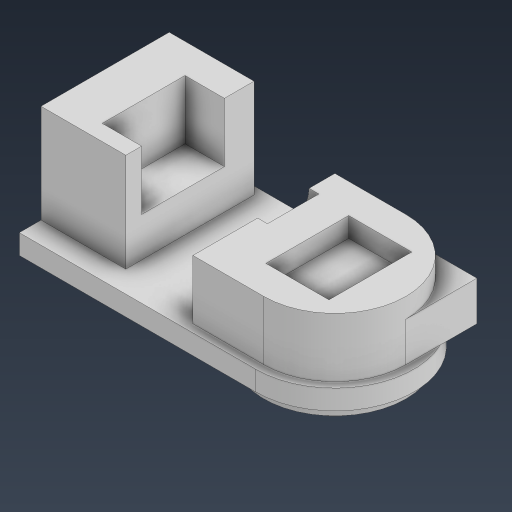
# Autodesk Inventor part: Axis1
Saved by Autodesk Inventor 2024 (Build 280153000, 153)
## iProperties
Created: 2025-08-29
Part Number: Axis1
Material: Generic
Document SubType Name: Modeling
Designer: Piter
Density: 1 g/cm^3
Appearance: Default
Author: Piter
Autodesk Inventor part; units mm, degrees
ref_plane "YZ Plane" through (0, 0, 0) normal (1, 0, 0) x (0, 1, 0)
ref_plane "XZ Plane" through (0, 0, 0) normal (0, 1, 0) x (-1, 0, 0)
sketch "Sketch1" plane through (0, 0, 0) normal (0, 1, 0) x (-1, 0, 0)
  circle A0 centre (0, 0) radius 19.95
  dimension "d0" = 39.9
  constraints: 1 centre point, 1 coincident
  measures "d0" diameter of A0
extrude "Extrusion1" add sketch "Sketch1" along normal blind 11.5
sketch "Sketch3" plane through (0, 11.5, 0) normal (0, 1, 0) x (1, 0, 0)
  circle A0 centre (0, 0) radius 36
  dimension "d4" = 72
  constraints: 1 centre point, 1 coincident
  measures "d4" diameter of A0
extrude "Extrusion2" add sketch "Sketch3" along normal blind 5
sketch "Sketch5" plane through (0, 0, 0) normal (0, -1, 0) x (1, 0, 0)
  circle A0 centre (0, 0) radius 12
  dimension "d10" = 24
  constraints: 1 centre point, 1 coincident
  measures "d10" diameter of A0
extrude "Extrusion4" add sketch "Sketch5" along normal blind 4
sketch "Sketch6" plane through (0, -4, 0) normal (0, -1, 0) x (1, 0, 0)
  circle A0 centre (0, 0) radius 8
  dimension "d13" = 16
  constraints: 1 centre point, 1 coincident
  measures "d13" diameter of A0
extrude "Extrusion5" cut sketch "Sketch6" against normal blind 7
sketch "Sketch7" plane through (0, 0, 0) normal (0, 0, 1) x (1, 0, 0)
  line L0 (-12, -4) -> (12, -4) projected
  line L1 (0, -4) -> (0, 16.5) construction
  line L2 (36, 16.5) -> (-36, 16.5) projected
  circle A0 centre (0, -0.5) radius 2.05
  point P0 (0, 0)
  dimension "d16" = 4.1
  dimension "d17" = 3.5
  constraints: 2 end point, 2 midpoint, 1 centre point, 1 point on line
  measures "d16" diameter of A0
  measures "d17" distance from line of L0 A0.centre
extrude "Extrusion6" cut sketch "Sketch7" against normal through all
ref_plane "Work Plane1" through (0, 0, -9) normal (0, 0, 1) x (1, 0, 0)
sketch "Sketch8" plane through (0, 0, -9) normal (0, 0, 1) x (1, 0, 0)
  spline S0 degree 8 poles (2.05, -0.5) (2.05, -0.2848) (2.0242, -0.07) (1.9727, 0.1426) (1.8952, 0.3508) (1.7908, 0.5524) (1.6587, 0.744) (1.4975, 0.9217) (1.1428, 1.2152) (0.9502, 1.3418) (0.7319, 1.4481) (0.4932, 1.5258) (0.2416, 1.5696) (-0.015, 1.5768) (-0.268, 1.5477) (-0.7585, 1.4217) (-0.9865, 1.3253) (-1.1913, 1.203) (-1.372, 1.0604) (-1.5283, 0.9024) (-1.6604, 0.7329) (-1.769, 0.5554) (-1.9523, 0.1659) (-2.022, -0.0509) (-2.064, -0.2739) (-2.0779, -0.5) (-2.064, -0.7261) (-2.022, -0.9491) (-1.9523, -1.1659) (-1.7743, -1.544) (-1.674, -1.7105) (-1.5532, -1.8699) (-1.4114, -2.0197) (-1.2482, -2.1567) (-1.0637, -2.2771) (-0.8583, -2.3766) (-0.4199, -2.5191) (-0.1917, -2.5636) (0.0445, -2.5784) (0.2816, -2.5615) (0.512, -2.5135) (0.7285, -2.4379) (0.9254, -2.3407) (1.3434, -2.0754) (1.5505, -1.8884) (1.7199, -1.6798) (1.8532, -1.4566) (1.9518, -1.2237) (2.0171, -0.9848) (2.05, -0.7427) (2.05, -0.5) knots 0 0 0 0 0 0 0 0 0 0.154447 0.154447 0.154447 0.154447 0.154447 0.154447 0.154447 0.287129 0.287129 0.287129 0.287129 0.287129 0.287129 0.287129 0.423569 0.423569 0.423569 0.423569 0.423569 0.423569 0.423569 0.578272 0.578272 0.578272 0.578272 0.578272 0.578272 0.578272 0.706239 0.706239 0.706239 0.706239 0.706239 0.706239 0.706239 0.827838 0.827838 0.827838 0.827838 0.827838 0.827838 0.827838 1 1 1 1 1 1 1 1 1 projected
  line L0 (8, 3) -> (-8, 3) projected
  line L1 (8, -4) -> (-8, -4) projected
  circle A0 centre (0, -0.5) radius 3
  point P0 (0, 0)
  dimension "d21" = 6
  constraints: 1 centre point, 1 other
  measures "d21" diameter of A0
extrude "Extrusion7" cut sketch "Sketch8" against normal through all
pattern_circular "Circular Pattern1" count 2 over 90 about axis through (0, -10, 0) along (0, 1, 0) of "Extrusion7", "Extrusion6"
sketch "Sketch10" plane through (0, 16.5, 0) normal (0, 1, 0) x (1, 0, 0)
  circle A0 centre (0, 0) radius 36 projected
  circle A1 centre (0, 0) radius 40
  line L0 (0, 40) -> (0, -40)
  line L1 (0, -40) -> (-70, -40)
  line L2 (-70, -40) -> (-70, 40)
  line L3 (-70, 40) -> (0, 40)
  dimension "d51" = 80
  dimension "d67" = 70
  constraints: 8 end point, 2 parallel, 2 point on circle, 1 centre point, 1 coincident, 1 perpendicular
  measures "d51" diameter of A1
  measures "d67" distance of L0.end L1.end
extrude "Extrusion8" add sketch "Sketch10" along normal blind 10 contours A0 L0 | A0 L0 A1 | L0 A0 | A0 L0 A1
sketch "Sketch11" plane through (0, 26.5, 0) normal (0, 1, 0) x (1, 0, 0)
  line L0 (-36, -36) -> (36, -36)
  line L1 (36, -36) -> (36, 36)
  line L2 (36, 36) -> (-36, 36)
  line L3 (-36, 36) -> (-36, -36)
  circle A0 centre (0, 0) radius 8 projected
  line L4 (-36, -36) -> (36, 36) construction
  line L5 (36, -36) -> (-36, 36) construction
  line L6 (0, 36) -> (0, -36) construction
  line L7 (-36, 0) -> (36, 0) construction
  circle A1 centre (0, 0) radius 36 projected
  line L8 (-14, -21) -> (18, -21)
  line L9 (18, -21) -> (18, 21)
  line L10 (18, 21) -> (-14, 21)
  line L11 (-14, 21) -> (-14, -21)
  line L12 (-14, -21) -> (18, 21) construction
  line L13 (18, -21) -> (-14, 21) construction
  circle A2 centre (0, 0) radius 40 projected
  line L14 (18, 21) -> (18, 35.7211)
  line L15 (18, -21) -> (18, -35.7211)
  line L16 (18, 35.7211) -> (18, -35.7211)
  line L17 (18, -35.7211) -> (-34, -35.7211)
  line L18 (-34, -35.7211) -> (-34, 35.7211)
  line L19 (-34, 35.7211) -> (18, 35.7211)
  line L20 (-14, 0) -> (-36, 0)
  line L21 (18, -29) -> (-21.3307, -29)
  point P0 (2, 0)
  point P1 (-18, 35.7211)
  point P2 (-36, 29.3939)
  point P3 (-36, -29.3939)
  point P4 (-18, -35.7211)
  point P5 (6, -5.2915)
  point P6 (6, 5.2915)
  point P7 (6, 36)
  point P8 (6, -36)
  point P9 (18, -29)
  point P10 (18, 31.1769)
  point P11 (18, -31.1769)
  dimension "d35" = 72
  dimension "d36" = 72
  dimension "d37" = 32
  dimension "d38" = 42
  dimension "d39" = 18
  dimension "d40" = 52
  dimension "d53" = 7
  constraints: 44 end point, 9 midpoint, 6 parallel, 4 perpendicular, 4 point on circle, 3 point on line, 2 horizontal, 1 collinear, 1 vertical
  measures "d35" distance of L2.end L1.end
  measures "d36" distance of L1.end L0.end
  measures "d37" distance of L10.end L9.end
  measures "d38" distance of L9.end L8.end
  measures "d39" distance between parallel lines of L1 L9
  measures "d40" distance of L15.end L17.end
  measures "d53" distance between parallel lines of L0 L21
extrude "Extrusion9" add sketch "Sketch11" along normal blind 20 contours L3 A2 L18 L17 L0 | A2 L17 A1 L0 | L3 A1 L18 A2 | A1 L17 A2 L0 | A1 L17 | L17 L18 A2 | A2 L18 A1 L17 | A2 L1 L0 | L3 A2 L18 A1 | L20 L18 A1 | A1 L18 L20 | L3 L2 A2 L19 L18 | A1 L21 L15 L17 | A1 L15 L17 | L15 A1 L1 A2 | L18 A2 L19 A1 | A1 L19 L14 L10 L11 L20 L18 | L18 L20 L11 L8 L15 L21 A1 | L18 L19 A2 | L15 L9 L14 A1 | L19 A2 L2 A1 | A1 L19 | L11 L10 L9 L8 | A1 L14 A2 L1 | L2 A2 L19 A1 | L19 L14 A1 | L2 L1 A2 | A0
extrude "Extrusion10" add sketch "Sketch11" along normal blind 30 contours L3 A2 L18 L17 L0 | A2 L17 A1 L0 | L3 A1 L18 A2 | A1 L17 | L17 L18 A2 | A2 L18 A1 L17 | L3 A2 L18 A1 | L20 L18 A1 | A1 L18 L20 | L3 L2 A2 L19 L18 | A1 L21 L15 L17 | L18 A2 L19 A1 | A1 L19 L14 L10 L11 L20 L18 | L18 L20 L11 L8 L15 L21 A1 | L18 L19 A2 | L15 L9 L14 A1 | L19 A2 L2 A1 | A1 L19 picked at (-8.298, -35.8657) picked at (-8.298, 35.8657)
sketch "Sketch15" plane through (0, 46.5, 0) normal (0, 1, 0) x (1, 0, 0)
  arc A0 (0, -36) -> (36, 0) centre (0, 0) ccw projected
  line L0 (0, -36) -> (36, -36) projected
  line L1 (36, -36) -> (36, 0) projected
  arc A1 (36, 0) -> (0, 36) centre (0, 0) ccw projected
  line L2 (36, 0) -> (36, 36) projected
  line L3 (36, 36) -> (0, 36) projected
extrude "Extrusion12" cut sketch "Sketch15" against normal up to surface (20 mm away) contours A0 L1 L0
sketch "Sketch16" plane through (0, 56.5, 0) normal (0, 1, 0) x (1, 0, 0)
  line L0 (-14, -21) -> (-14, 21) projected
  line L1 (18, -21) -> (-14, -21) projected
  line L2 (-14, -21) -> (-14, 21) projected
  line L3 (-14, 21) -> (18, 21) projected
  line L4 (0, 36) -> (-36, 36) projected
  line L5 (-36, 36) -> (-36, -36) projected
  arc A0 (0, -36) -> (0, 36) centre (0, 0) ccw projected
  line L6 (-34.5832, -10) -> (-14, -10)
  line L7 (-14, 36) -> (-14, 21)
  line L8 (-36, -36) -> (0, -36) projected
  line L9 (18, 21) -> (18, -21) projected
  point P0 (-14, 21)
  constraints: 4 end point, 2 point on line, 1 collinear, 1 horizontal, 1 point on circle
extrude "Extrusion13" add sketch "Sketch16" along normal blind 15 contours L0 L3 L9 L1 | A0 L8 L5 L4
sketch "Sketch17" plane through (-36, 26.5, -36) normal (-1, 0, 0) x (0, 0, 1)
  line L0 (0, 45) -> (72, 45) projected
  line L1 (0, 0) -> (0, 45) projected
  line L2 (0, 0) -> (18.5644, 0) projected
  line L3 (53.4356, 0) -> (18.5644, 0) projected
  line L4 (15, 20) -> (57, 20) projected
  line L5 (15, 20) -> (15, 30) projected
  circle A0 centre (26.14, 30.25) radius 13.05
  line L6 (53.4356, 0) -> (72, 0) projected
  line L7 (72, 0) -> (72, 45) projected
  point P0 (36, -26.5)
  dimension "d59" = 26.1
  dimension "d60" = 10.25
  dimension "d61" = 11.14
  constraints: 1 centre point
  measures "d59" diameter of A0
  measures "d60" distance from line of L4 A0.centre
  measures "d61" distance from line of A0.centre L5
extrude "Extrusion14" cut sketch "Sketch17" against normal blind 5 contours A0 L4 | L4 A0
sketch "Sketch18" plane through (0, 71.5, 0) normal (0, 1, 0) x (1, 0, 0)
  arc A0 (0, -36) -> (0, 36) centre (0, 0) ccw projected
  line L0 (0, 36) -> (-36, 36) projected
  line L1 (-36, 36) -> (-36, -36) projected
  line L2 (-31, -3.19) -> (-31, 22.91) projected
  line L3 (-26, -9.6438) -> (-34.6842, -9.6438)
  line L4 (-36, -36) -> (0, -36) projected
  constraints: 2 end point, 1 horizontal, 1 point on circle
extrude "Extrusion15" cut sketch "Sketch18" against normal blind 15
sketch "Sketch19" plane through (0, 26.5, 0) normal (0, 1, 0) x (1, 0, 0)
  arc A0 (-36, 17.4356) -> (-36, -17.4356) centre (0, 0) ccw projected
  line L0 (-17.4356, 36) -> (17.4356, 36) projected
  arc A1 (0, -36) -> (36, 0) centre (0, 0) ccw projected
  line L1 (-36, -17.4356) -> (-36, 17.4356) projected
  line L2 (0, -40) -> (0, 40)
  line L3 (0, 40) -> (-120, 40)
  line L4 (-120, 40) -> (-120, -40)
  line L5 (-120, -40) -> (0, -40)
  line L6 (-77, 21) -> (-109, 21)
  line L7 (-109, 21) -> (-109, -21)
  line L8 (-109, -21) -> (-77, -21)
  line L9 (-77, -21) -> (-77, 21)
  line L10 (18, 21) -> (-14, 21) construction
  line L11 (-14, 21) -> (-14, -21) construction
  line L12 (-14, -21) -> (18, -21) construction
  line L13 (-14, 21) -> (18, 21) construction
  line L14 (18, -21) -> (18, 21) projected
  line L15 (0, -36) -> (-17.4356, -36) projected
  arc A2 (-17.4356, -36) -> (36, 17.4356) centre (0, 0) ccw projected
  line L16 (36, 17.4356) -> (36, 0) projected
  arc A3 (17.4356, 36) -> (-17.4356, 36) centre (0, 0) ccw projected
  point P0 (0, 36)
  dimension "d68" = 120
  dimension "d71" = 42
  dimension "d72" = 32
  constraints: 16 end point, 4 parallel, 2 perpendicular, 2 point on circle, 1 collinear, 1 horizontal, 1 vertical
  measures "d68" distance of L3.end L2.end
  measures "d71" distance of L7.end L6.end
  measures "d72" distance of L7.end L8.end
extrude "Extrusion16" add sketch "Sketch19" against normal blind 10 contours A3 L2 L0 | L0 L2 L15 A2 L5 L4 L3 A3 | L2 A3 L0 | L2 A2 L15 | L9 L8 L7 L6
sketch "Sketch20" plane through (0, 26.5, 0) normal (0, 1, 0) x (1, 0, 0)
  line L0 (-36, 36) -> (17.4356, 36) projected
  arc A0 (0, -36) -> (36, 0) centre (0, 0) ccw projected
  line L1 (-36, 36) -> (-36, -36) projected
  line L2 (0, 40) -> (-120, 40) projected
  line L3 (-120, 40) -> (-120, -40) projected
  line L4 (-120, -40) -> (0, -40) projected
  arc A1 (0, -40) -> (36, 17.4356) centre (0, 0) ccw projected
  line L5 (-77, 21) -> (-77, 36)
  line L6 (-77, 36) -> (-120, 36)
  line L7 (-77, -21) -> (-77, -29)
  line L8 (-77, -29) -> (-120, -29)
  line L9 (6, -29) -> (-17.0441, -29) projected
  line L10 (6, 36) -> (-26, 36) projected
  line L11 (-77, 21) -> (-77, -21)
  line L12 (-77, -21) -> (-97, -21)
  line L13 (-97, -21) -> (-97, 21)
  line L14 (-97, 21) -> (-77, 21)
  line L15 (36, 17.4356) -> (36, 0) projected
  line L16 (-36, -36) -> (0, -36) projected
  arc A2 (17.4356, 36) -> (0, 40) centre (0, 0) ccw projected
  dimension "d74" = 20
  dimension "d75" = 41
  dimension "d76" = 42
  constraints: 16 end point, 4 perpendicular, 3 collinear, 3 point on line, 1 horizontal, 1 vertical
  measures "d74" distance of L7.start L12.end
  measures "d75" distance between parallel lines of L1 L11
  measures "d76" distance of L12.end L13.end
extrude "Extrusion17" add sketch "Sketch20" along normal blind 20 contours L6 L5 L14 L13 L12 L7 L8 L3 | L11 L12 L13 L14
extrude "Extrusion18" add sketch "Sketch20" along normal blind 50 contours L6 L5 L14 L13 L12 L7 L8 L3
body "Solid1"
